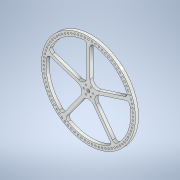
# Autodesk Inventor part: spokes
Saved by Autodesk Inventor 2022.2 (Build 262287000, 287)
## iProperties
Created: 2021-11-12
Part Number: spokes
Material: Generic
Document SubType Name: Modeling
Designer: gnzak
Density: 1 g/cm^3
Appearance: Default
Autodesk Inventor part; units mm, degrees
ref_plane "YZ Plane" through (0, 0, 0) normal (1, 0, 0) x (0, 1, 0)
ref_plane "XZ Plane" through (0, 0, 0) normal (0, 1, 0) x (-1, 0, 0)
ref_plane "XY Plane" through (0, 0, 0) normal (0, 0, 1) x (1, 0, 0)
sketch "Sketch1" plane through (0, 0, 0) normal (0, 0, 1) x (1, 0, 0)
  point P0 (0, 0)
sketch "0" plane through (0, 0, 0) normal (0, 0, 1) x (1, 0, 0)
  line L0 (21.7618, 3.7324) -> (75.9257, 21.3314)
  arc A0 (84.119, 16.5155) -> (75.9257, 21.3314) centre (77.888, 15.2922) ccw
  arc A1 (58.3461, -62.8053) -> (84.119, 16.5155) centre (0, 0) ccw
  arc A2 (48.8869, -61.8855) -> (58.3461, -62.8053) centre (54.0242, -58.153) ccw
  line L1 (48.8869, -61.8855) -> (15.4118, -15.8109)
  arc A3 (21.7618, 3.7324) -> (15.4118, -15.8109) centre (25.6863, -8.346) ccw
  line L2 (10.2745, -19.5433) -> (43.7497, -65.6179)
  arc A4 (41.7014, -74.8984) -> (43.7497, -65.6179) centre (38.6124, -69.3503) ccw
  arc A5 (-41.7014, -74.8984) -> (41.7014, -74.8984) centre (0, 0) ccw
  arc A6 (-43.7497, -65.6179) -> (-41.7014, -74.8984) centre (-38.6124, -69.3503) ccw
  line L3 (-43.7497, -65.6179) -> (-10.2745, -19.5433)
  arc A7 (10.2745, -19.5433) -> (-10.2745, -19.5433) centre (0, -27.0082) ccw
  line L4 (-15.4118, -15.8109) -> (-48.8869, -61.8855)
  arc A8 (-58.3461, -62.8053) -> (-48.8869, -61.8855) centre (-54.0242, -58.153) ccw
  arc A9 (-84.119, 16.5155) -> (-58.3461, -62.8053) centre (0, 0) ccw
  arc A10 (-75.9257, 21.3314) -> (-84.119, 16.5155) centre (-77.888, 15.2922) ccw
  line L5 (-75.9257, 21.3314) -> (-21.7618, 3.7324)
  arc A11 (-15.4118, -15.8109) -> (-21.7618, 3.7324) centre (-25.6863, -8.346) ccw
  line L6 (-19.7995, 9.7716) -> (-73.9635, 27.3706)
  arc A12 (-77.7613, 36.0826) -> (-73.9635, 27.3706) centre (-72.0012, 33.4098) ccw
  arc A13 (-10.287, 85.1055) -> (-77.7613, 36.0826) centre (0, 0) ccw
  arc A14 (-3.175, 78.8014) -> (-10.287, 85.1055) centre (-9.525, 78.8014) ccw
  line L7 (-3.175, 78.8014) -> (-3.175, 21.8501)
  arc A15 (-19.7995, 9.7716) -> (-3.175, 21.8501) centre (-15.875, 21.8501) ccw
  arc A16 (77.7613, 36.0826) -> (10.287, 85.1055) centre (0, 0) ccw
  arc A17 (73.9635, 27.3706) -> (77.7613, 36.0826) centre (72.0012, 33.4098) ccw
  line L8 (73.9635, 27.3706) -> (19.7995, 9.7716)
  arc A18 (3.175, 21.8501) -> (19.7995, 9.7716) centre (15.875, 21.8501) ccw
  line L9 (3.175, 21.8501) -> (3.175, 78.8014)
  arc A19 (10.287, 85.1055) -> (3.175, 78.8014) centre (9.525, 78.8014) ccw
  circle A20 centre (0, 0) radius 3.175
  circle A21 centre (7.0996, 90.2086) radius 1.6724
  circle A22 centre (14.1554, 89.3734) radius 1.6724
  circle A23 centre (21.1239, 87.9873) radius 1.6724
  circle A24 centre (27.9622, 86.0587) radius 1.6724
  circle A25 centre (34.6281, 83.5995) radius 1.6724
  circle A26 centre (41.0805, 80.625) radius 1.6724
  circle A27 centre (47.2796, 77.1533) radius 1.6724
  circle A28 centre (53.1872, 73.2059) radius 1.6724
  circle A29 centre (58.7669, 68.8072) radius 1.6724
  circle A30 centre (63.9843, 63.9843) radius 1.6724
  circle A31 centre (68.8072, 58.7669) radius 1.6724
  circle A32 centre (73.2059, 53.1872) radius 1.6724
  circle A33 centre (77.1533, 47.2796) radius 1.6724
  circle A34 centre (80.625, 41.0805) radius 1.6724
  circle A35 centre (83.5995, 34.6281) radius 1.6724
  circle A36 centre (86.0587, 27.9622) radius 1.6724
  circle A37 centre (87.9873, 21.1239) radius 1.6724
  circle A38 centre (89.3734, 14.1554) radius 1.6724
  circle A39 centre (90.2086, 7.0996) radius 1.6724
  circle A40 centre (90.4875, 0) radius 1.6724
  circle A41 centre (90.2086, -7.0996) radius 1.6724
  circle A42 centre (89.3734, -14.1554) radius 1.6724
  circle A43 centre (87.9873, -21.1239) radius 1.6724
  circle A44 centre (86.0587, -27.9622) radius 1.6724
  circle A45 centre (83.5995, -34.6281) radius 1.6724
  circle A46 centre (80.625, -41.0805) radius 1.6724
  circle A47 centre (77.1533, -47.2796) radius 1.6724
  circle A48 centre (73.2059, -53.1872) radius 1.6724
  circle A49 centre (68.8072, -58.7669) radius 1.6724
  circle A50 centre (63.9843, -63.9843) radius 1.6724
  circle A51 centre (58.7669, -68.8072) radius 1.6724
  circle A52 centre (53.1872, -73.2059) radius 1.6724
  circle A53 centre (47.2796, -77.1533) radius 1.6724
  circle A54 centre (41.0805, -80.625) radius 1.6724
  circle A55 centre (34.6281, -83.5995) radius 1.6724
  circle A56 centre (27.9622, -86.0587) radius 1.6724
  circle A57 centre (21.1239, -87.9873) radius 1.6724
  circle A58 centre (14.1554, -89.3734) radius 1.6724
  circle A59 centre (7.0996, -90.2086) radius 1.6724
  circle A60 centre (0, -90.4875) radius 1.6724
  circle A61 centre (-7.0996, -90.2086) radius 1.6724
  circle A62 centre (-14.1554, -89.3734) radius 1.6724
  circle A63 centre (-21.1239, -87.9873) radius 1.6724
  circle A64 centre (-27.9622, -86.0587) radius 1.6724
  circle A65 centre (-34.6281, -83.5995) radius 1.6724
  circle A66 centre (-41.0805, -80.625) radius 1.6724
  circle A67 centre (-47.2796, -77.1533) radius 1.6724
  circle A68 centre (-53.1872, -73.2059) radius 1.6724
  circle A69 centre (-58.7669, -68.8072) radius 1.6724
  circle A70 centre (-63.9843, -63.9843) radius 1.6724
  circle A71 centre (-68.8072, -58.7669) radius 1.6724
  circle A72 centre (-73.2059, -53.1872) radius 1.6724
  circle A73 centre (-77.1533, -47.2796) radius 1.6724
  circle A74 centre (-80.625, -41.0805) radius 1.6724
  circle A75 centre (-83.5995, -34.6281) radius 1.6724
  circle A76 centre (-86.0587, -27.9622) radius 1.6724
  circle A77 centre (-87.9873, -21.1239) radius 1.6724
  circle A78 centre (-89.3734, -14.1554) radius 1.6724
  circle A79 centre (-90.2086, -7.0996) radius 1.6724
  circle A80 centre (-90.4875, 0) radius 1.6724
  circle A81 centre (-90.2086, 7.0996) radius 1.6724
  circle A82 centre (-89.3734, 14.1554) radius 1.6724
  circle A83 centre (-87.9873, 21.1239) radius 1.6724
  circle A84 centre (-86.0587, 27.9622) radius 1.6724
  circle A85 centre (-83.5995, 34.6281) radius 1.6724
  circle A86 centre (-80.625, 41.0805) radius 1.6724
  circle A87 centre (-77.1533, 47.2796) radius 1.6724
  circle A88 centre (-73.2059, 53.1872) radius 1.6724
  circle A89 centre (-68.8072, 58.7669) radius 1.6724
  circle A90 centre (-63.9843, 63.9843) radius 1.6724
  circle A91 centre (-58.7669, 68.8072) radius 1.6724
  circle A92 centre (-53.1872, 73.2059) radius 1.6724
  circle A93 centre (-47.2796, 77.1533) radius 1.6724
  circle A94 centre (-41.0805, 80.625) radius 1.6724
  circle A95 centre (-34.6281, 83.5995) radius 1.6724
  circle A96 centre (-27.9622, 86.0587) radius 1.6724
  circle A97 centre (-21.1239, 87.9873) radius 1.6724
  circle A98 centre (-14.1554, 89.3734) radius 1.6724
  circle A99 centre (-7.0996, 90.2086) radius 1.6724
  circle A100 centre (0, 90.4875) radius 1.6724
  circle A101 centre (4.7625, -8.2489) radius 1.4224
  circle A102 centre (-4.7625, -8.2489) radius 1.4224
  circle A103 centre (-9.525, 0) radius 1.4224
  circle A104 centre (-4.7625, 8.2489) radius 1.4224
  circle A105 centre (4.7625, 8.2489) radius 1.4224
  circle A106 centre (9.525, 0) radius 1.4224
  circle A107 centre (0, 0) radius 95.25
  point P0 (19.7995, 9.7716)
  point P1 (3.175, 21.8501)
  point P2 (10.287, 85.1055)
  point P3 (-3.175, 78.8014)
  point P4 (-3.175, 21.8501)
  point P5 (-21.7618, 3.7324)
  point P6 (-48.8869, -61.8855)
  point P7 (41.7014, -74.8984)
  point P8 (-41.7014, -74.8984)
  point P9 (15.4118, -15.8109)
  point P10 (75.9257, 21.3314)
  point P11 (58.3461, -62.8053)
  constraints: 108 centre point, 40 point on circle, 20 end point
extrude "Extrusion1" add sketch "0" along normal blind 6.35
body "Solid1"
